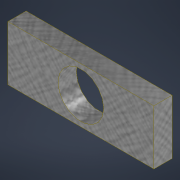
# Autodesk Inventor part: McCrea_doska_walle
Saved by Autodesk Inventor 2022 (Build 260153000, 153)
## iProperties
Created: 2022-02-06
Part Number: McCrea_doska_walle
Material: Silver
Document SubType Name: Modeling
Designer: Max
Density: 10.49 g/cm^3
Appearance: Silver
Author: Max
Autodesk Inventor part; units mm, degrees
ref_plane "YZ Plane" through (0, 0, 0) normal (1, 0, 0) x (0, 1, 0)
ref_plane "XZ Plane" through (0, 0, 0) normal (0, 1, 0) x (-1, 0, 0)
ref_plane "XY Plane" through (0, 0, 0) normal (0, 0, 1) x (1, 0, 0)
sketch "Sketch1" plane through (0, 0, 0) normal (0, 0, 1) x (1, 0, 0)
  line L0 (-11.9806, 5.9141) -> (-3.9806, 5.9141)
  line L1 (-3.9806, 5.9141) -> (-3.9806, 2.9141)
  line L2 (-3.9806, 2.9141) -> (-11.9806, 2.9141)
  line L3 (-11.9806, 2.9141) -> (-11.9806, 5.9141)
  circle A0 centre (-7.9806, 4.4141) radius 1.25
  point P0 (0, 0)
  dimension "d0" = 8
  dimension "d1" = 3
  dimension "d11" = 2.5
  dimension "d12" = 1.5
  dimension "d13" = 4
  constraints: 8 end point, 2 parallel, 1 centre point, 1 horizontal, 1 perpendicular
  measures "d0" distance of L1.end L2.end
  measures "d1" distance of L2.end L0.start
  measures "d11" diameter of A0
  measures "d12" distance from line of L0 A0.centre
  measures "d13" distance from line of L3 A0.centre
extrude "Extrusion1" add sketch "Sketch1" along normal blind 1 contours L0 L1 L2 L3 | A0
hole "Hole2" at (-7.9806, 4.4141, 0) direction (0, 0, 1) diameter 2.5 depth 3 tip angle 118
body "Solid1"
